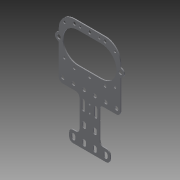
# Autodesk Inventor part: xcarriage
Saved by Autodesk Inventor 2014 (Build 180170000, 170)
## iProperties
Created: 2013-12-23
Part Number: xcarriage
Material: Generic
Document SubType Name: Modeling
Designer: stephen
Density: 1 g/cm^3
Appearance: Default
Author: stephen
Autodesk Inventor part; units mm, degrees
ref_plane "YZ Plane" through (0, 0, 0) normal (1, 0, 0) x (0, 1, 0)
ref_plane "XZ Plane" through (0, 0, 0) normal (0, 1, 0) x (-1, 0, 0)
ref_plane "XY Plane" through (0, 0, 0) normal (0, 0, 1) x (1, 0, 0)
sketch "Sketch1" plane through (0, 0, 0) normal (0, 1, 0) x (-1, 0, 0)
  line L0 (191.3405, 93.7812) -> (191.3405, 90.7812)
  circle A0 centre (230.8405, 152.2812) radius 2.5
  arc A1 (154.4119, 200.0727) -> (155.8405, 201.9894) centre (153.8405, 201.9894) ccw
  line L1 (200.3405, 110.7812) -> (200.3405, 113.7812)
  line L2 (186.3405, 90.7812) -> (186.3405, 93.7812)
  circle A2 centre (216.8405, 152.2812) radius 2.5
  arc A3 (213.8405, 145.2812) -> (208.8405, 140.2812) centre (213.8405, 140.2812) ccw
  line L3 (180.8405, 175.2812) -> (210.8405, 175.2812)
  arc A4 (182.8405, 127.2812) -> (182.8458, 127.0511) centre (187.8405, 127.2812) ccw
  line L4 (210.8405, 215.2812) -> (180.8405, 215.2812)
  arc A5 (201.8405, 129.2812) -> (205.8405, 129.2812) centre (203.8405, 129.2812) ccw
  arc A6 (154.4119, 200.0727) -> (154.4119, 190.4896) centre (155.8405, 195.2812) ccw
  line L5 (219.3405, 93.7812) -> (219.3405, 90.7812)
  line L6 (217.3405, 99.7812) -> (213.8405, 99.7812)
  arc A7 (214.3405, 90.7812) -> (219.3405, 90.7812) centre (216.8405, 90.7812) ccw
  line L7 (208.8405, 104.7812) -> (208.8405, 127.0511)
  arc A8 (200.3405, 110.7812) -> (205.3405, 110.7812) centre (202.8405, 110.7812) ccw
  circle A9 centre (215.8405, 220.2812) radius 2.1
  circle A10 centre (160.8405, 152.2812) radius 2.5
  arc A11 (191.3405, 93.7812) -> (186.3405, 93.7812) centre (188.8405, 93.7812) ccw
  line L8 (182.8405, 127.0511) -> (182.8405, 104.7812)
  arc A12 (169.3405, 89.7812) -> (174.3405, 84.7812) centre (174.3405, 89.7812) ccw
  circle A13 centre (215.8405, 170.2812) radius 2.1
  line L9 (175.8405, 225.2812) -> (215.8405, 225.2812)
  arc A14 (217.3405, 84.7812) -> (222.3405, 89.7812) centre (217.3405, 89.7812) ccw
  arc A15 (186.3405, 110.7812) -> (191.3405, 110.7812) centre (188.8405, 110.7812) ccw
  line L10 (205.3405, 93.7812) -> (205.3405, 90.7812)
  line L11 (186.3405, 110.7812) -> (186.3405, 113.7812)
  arc A16 (237.2691, 190.4896) -> (235.8405, 188.573) centre (237.8405, 188.573) ccw
  line L12 (177.3405, 93.7812) -> (177.3405, 90.7812)
  arc A17 (191.3405, 113.7812) -> (186.3405, 113.7812) centre (188.8405, 113.7812) ccw
  line L13 (189.8405, 129.2812) -> (189.8405, 139.2812)
  line L14 (235.8405, 188.573) -> (235.8405, 150.2812)
  circle A18 centre (175.8405, 170.2812) radius 2.1
  line L15 (172.3405, 90.7812) -> (172.3405, 93.7812)
  line L16 (174.3405, 84.7812) -> (217.3405, 84.7812)
  arc A19 (172.3405, 90.7812) -> (177.3405, 90.7812) centre (174.8405, 90.7812) ccw
  circle A20 centre (183.3405, 220.2812) radius 1.6
  line L17 (185.8405, 139.2812) -> (185.8405, 129.2812)
  arc A21 (222.3405, 94.7812) -> (217.3405, 99.7812) centre (217.3405, 94.7812) ccw
  arc A22 (200.3405, 90.7812) -> (205.3405, 90.7812) centre (202.8405, 90.7812) ccw
  line L18 (155.8405, 150.2812) -> (155.8405, 188.573)
  arc A23 (235.8405, 205.2812) -> (215.8405, 225.2812) centre (215.8405, 205.2812) ccw
  arc A24 (155.8405, 188.573) -> (154.4119, 190.4896) centre (153.8405, 188.573) ccw
  line L19 (222.3405, 89.7812) -> (222.3405, 94.7812)
  arc A25 (185.8405, 129.2812) -> (189.8405, 129.2812) centre (187.8405, 129.2812) ccw
  circle A26 centre (155.8405, 195.2812) radius 2.6
  line L20 (160.8405, 145.2812) -> (177.8405, 145.2812)
  arc A27 (177.3405, 93.7812) -> (172.3405, 93.7812) centre (174.8405, 93.7812) ccw
  arc A28 (186.3405, 90.7812) -> (191.3405, 90.7812) centre (188.8405, 90.7812) ccw
  circle A29 centre (202.8405, 152.2812) radius 2.5
  arc A30 (182.8405, 140.2812) -> (177.8405, 145.2812) centre (177.8405, 140.2812) ccw
  circle A31 centre (174.8405, 152.2812) radius 2.5
  line L21 (235.8405, 205.2812) -> (235.8405, 201.9894)
  line L22 (155.8405, 201.9894) -> (155.8405, 205.2812)
  line L23 (201.8405, 139.2812) -> (201.8405, 129.2812)
  circle A32 centre (162.8405, 215.2812) radius 1.75
  line L24 (208.8405, 127.0511) -> (208.8352, 127.0511)
  arc A33 (237.2691, 190.4896) -> (237.2691, 200.0727) centre (235.8405, 195.2812) ccw
  circle A34 centre (208.3405, 220.2812) radius 1.6
  arc A35 (208.8405, 104.7812) -> (213.8405, 99.7812) centre (213.8405, 104.7812) ccw
  arc A36 (189.8405, 139.2812) -> (185.8405, 139.2812) centre (187.8405, 139.2812) ccw
  arc A37 (219.3405, 93.7812) -> (214.3405, 93.7812) centre (216.8405, 93.7812) ccw
  line L25 (169.3405, 94.7812) -> (169.3405, 89.7812)
  circle A38 centre (228.8405, 175.2812) radius 1.75
  arc A39 (210.8405, 175.2812) -> (210.8405, 215.2812) centre (210.8405, 195.2812) ccw
  arc A40 (208.8352, 127.0511) -> (208.8405, 127.2812) centre (203.8405, 127.2812) ccw
  arc A41 (205.3405, 113.7812) -> (200.3405, 113.7812) centre (202.8405, 113.7812) ccw
  circle A42 centre (188.8405, 152.2812) radius 2.5
  arc A43 (174.3405, 99.7812) -> (169.3405, 94.7812) centre (174.3405, 94.7812) ccw
  circle A44 centre (195.8405, 220.2812) radius 2.1
  arc A45 (235.8405, 201.9894) -> (237.2691, 200.0727) centre (237.8405, 201.9894) ccw
  arc A46 (205.8405, 139.2812) -> (201.8405, 139.2812) centre (203.8405, 139.2812) ccw
  arc A47 (205.3405, 93.7812) -> (200.3405, 93.7812) centre (202.8405, 93.7812) ccw
  line L26 (208.8405, 127.2812) -> (208.8405, 140.2812)
  line L27 (182.8405, 127.2812) -> (182.8405, 140.2812)
  arc A48 (155.8405, 150.2812) -> (160.8405, 145.2812) centre (160.8405, 150.2812) ccw
  line L28 (200.3405, 90.7812) -> (200.3405, 93.7812)
  line L29 (182.8458, 127.0511) -> (182.8405, 127.0511)
  circle A49 centre (195.8405, 170.2812) radius 2.1
  arc A50 (180.8405, 215.2812) -> (180.8405, 175.2812) centre (180.8405, 195.2812) ccw
  line L30 (205.3405, 113.7812) -> (205.3405, 110.7812)
  line L31 (205.8405, 129.2812) -> (205.8405, 139.2812)
  line L32 (177.8405, 99.7812) -> (174.3405, 99.7812)
  circle A51 centre (235.8405, 195.2812) radius 2.6
  circle A52 centre (195.8405, 129.2812) radius 1.25
  line L33 (191.3405, 113.7812) -> (191.3405, 110.7812)
  arc A53 (175.8405, 225.2812) -> (155.8405, 205.2812) centre (175.8405, 205.2812) ccw
  circle A54 centre (162.8405, 175.2812) radius 1.75
  arc A55 (230.8405, 145.2812) -> (235.8405, 150.2812) centre (230.8405, 150.2812) ccw
  arc A56 (177.8405, 99.7812) -> (182.8405, 104.7812) centre (177.8405, 104.7812) ccw
  circle A57 centre (228.8405, 215.2812) radius 1.75
  circle A58 centre (175.8405, 220.2812) radius 2.1
  line L34 (213.8405, 145.2812) -> (230.8405, 145.2812)
  line L35 (214.3405, 90.7812) -> (214.3405, 93.7812)
  circle A59 centre (195.8405, 139.2812) radius 1.25
  line L36 (191.3405, 93.7812) -> (191.3405, 90.7812)
  circle A60 centre (230.8405, 152.2812) radius 2.5
  arc A61 (154.4119, 200.0727) -> (155.8405, 201.9894) centre (153.8405, 201.9894) ccw
  line L37 (200.3405, 110.7812) -> (200.3405, 113.7812)
  line L38 (186.3405, 90.7812) -> (186.3405, 93.7812)
  circle A62 centre (216.8405, 152.2812) radius 2.5
  arc A63 (213.8405, 145.2812) -> (208.8405, 140.2812) centre (213.8405, 140.2812) ccw
  line L39 (180.8405, 175.2812) -> (210.8405, 175.2812)
  arc A64 (182.8405, 127.2812) -> (182.8458, 127.0511) centre (187.8405, 127.2812) ccw
  line L40 (210.8405, 215.2812) -> (180.8405, 215.2812)
  arc A65 (201.8405, 129.2812) -> (205.8405, 129.2812) centre (203.8405, 129.2812) ccw
  arc A66 (154.4119, 200.0727) -> (154.4119, 190.4896) centre (155.8405, 195.2812) ccw
  line L41 (219.3405, 93.7812) -> (219.3405, 90.7812)
  line L42 (217.3405, 99.7812) -> (213.8405, 99.7812)
  arc A67 (214.3405, 90.7812) -> (219.3405, 90.7812) centre (216.8405, 90.7812) ccw
  line L43 (208.8405, 104.7812) -> (208.8405, 127.0511)
  arc A68 (200.3405, 110.7812) -> (205.3405, 110.7812) centre (202.8405, 110.7812) ccw
  circle A69 centre (215.8405, 220.2812) radius 2.1
  circle A70 centre (160.8405, 152.2812) radius 2.5
  arc A71 (191.3405, 93.7812) -> (186.3405, 93.7812) centre (188.8405, 93.7812) ccw
  line L44 (182.8405, 127.0511) -> (182.8405, 104.7812)
  arc A72 (169.3405, 89.7812) -> (174.3405, 84.7812) centre (174.3405, 89.7812) ccw
  circle A73 centre (215.8405, 170.2812) radius 2.1
  line L45 (175.8405, 225.2812) -> (215.8405, 225.2812)
  arc A74 (217.3405, 84.7812) -> (222.3405, 89.7812) centre (217.3405, 89.7812) ccw
  arc A75 (186.3405, 110.7812) -> (191.3405, 110.7812) centre (188.8405, 110.7812) ccw
  line L46 (205.3405, 93.7812) -> (205.3405, 90.7812)
  line L47 (186.3405, 110.7812) -> (186.3405, 113.7812)
  arc A76 (237.2691, 190.4896) -> (235.8405, 188.573) centre (237.8405, 188.573) ccw
  line L48 (177.3405, 93.7812) -> (177.3405, 90.7812)
  arc A77 (191.3405, 113.7812) -> (186.3405, 113.7812) centre (188.8405, 113.7812) ccw
  line L49 (189.8405, 129.2812) -> (189.8405, 139.2812)
  line L50 (235.8405, 188.573) -> (235.8405, 150.2812)
  circle A78 centre (175.8405, 170.2812) radius 2.1
  line L51 (172.3405, 90.7812) -> (172.3405, 93.7812)
  line L52 (174.3405, 84.7812) -> (217.3405, 84.7812)
  arc A79 (172.3405, 90.7812) -> (177.3405, 90.7812) centre (174.8405, 90.7812) ccw
  circle A80 centre (183.3405, 220.2812) radius 1.6
  line L53 (185.8405, 139.2812) -> (185.8405, 129.2812)
  arc A81 (222.3405, 94.7812) -> (217.3405, 99.7812) centre (217.3405, 94.7812) ccw
  arc A82 (200.3405, 90.7812) -> (205.3405, 90.7812) centre (202.8405, 90.7812) ccw
  line L54 (155.8405, 150.2812) -> (155.8405, 188.573)
  arc A83 (235.8405, 205.2812) -> (215.8405, 225.2812) centre (215.8405, 205.2812) ccw
  arc A84 (155.8405, 188.573) -> (154.4119, 190.4896) centre (153.8405, 188.573) ccw
  line L55 (222.3405, 89.7812) -> (222.3405, 94.7812)
  arc A85 (185.8405, 129.2812) -> (189.8405, 129.2812) centre (187.8405, 129.2812) ccw
  circle A86 centre (155.8405, 195.2812) radius 2.6
  line L56 (160.8405, 145.2812) -> (177.8405, 145.2812)
  arc A87 (177.3405, 93.7812) -> (172.3405, 93.7812) centre (174.8405, 93.7812) ccw
  arc A88 (186.3405, 90.7812) -> (191.3405, 90.7812) centre (188.8405, 90.7812) ccw
  circle A89 centre (202.8405, 152.2812) radius 2.5
  arc A90 (182.8405, 140.2812) -> (177.8405, 145.2812) centre (177.8405, 140.2812) ccw
  circle A91 centre (174.8405, 152.2812) radius 2.5
  line L57 (235.8405, 205.2812) -> (235.8405, 201.9894)
  line L58 (155.8405, 201.9894) -> (155.8405, 205.2812)
  line L59 (201.8405, 139.2812) -> (201.8405, 129.2812)
  circle A92 centre (162.8405, 215.2812) radius 1.75
  line L60 (208.8405, 127.0511) -> (208.8352, 127.0511)
  arc A93 (237.2691, 190.4896) -> (237.2691, 200.0727) centre (235.8405, 195.2812) ccw
  circle A94 centre (208.3405, 220.2812) radius 1.6
  arc A95 (208.8405, 104.7812) -> (213.8405, 99.7812) centre (213.8405, 104.7812) ccw
  arc A96 (189.8405, 139.2812) -> (185.8405, 139.2812) centre (187.8405, 139.2812) ccw
  arc A97 (219.3405, 93.7812) -> (214.3405, 93.7812) centre (216.8405, 93.7812) ccw
  line L61 (169.3405, 94.7812) -> (169.3405, 89.7812)
  circle A98 centre (228.8405, 175.2812) radius 1.75
  arc A99 (210.8405, 175.2812) -> (210.8405, 215.2812) centre (210.8405, 195.2812) ccw
  arc A100 (208.8352, 127.0511) -> (208.8405, 127.2812) centre (203.8405, 127.2812) ccw
  arc A101 (205.3405, 113.7812) -> (200.3405, 113.7812) centre (202.8405, 113.7812) ccw
  circle A102 centre (188.8405, 152.2812) radius 2.5
  arc A103 (174.3405, 99.7812) -> (169.3405, 94.7812) centre (174.3405, 94.7812) ccw
  circle A104 centre (195.8405, 220.2812) radius 2.1
  arc A105 (235.8405, 201.9894) -> (237.2691, 200.0727) centre (237.8405, 201.9894) ccw
  arc A106 (205.8405, 139.2812) -> (201.8405, 139.2812) centre (203.8405, 139.2812) ccw
  arc A107 (205.3405, 93.7812) -> (200.3405, 93.7812) centre (202.8405, 93.7812) ccw
  line L62 (208.8405, 127.2812) -> (208.8405, 140.2812)
  line L63 (182.8405, 127.2812) -> (182.8405, 140.2812)
  arc A108 (155.8405, 150.2812) -> (160.8405, 145.2812) centre (160.8405, 150.2812) ccw
  line L64 (200.3405, 90.7812) -> (200.3405, 93.7812)
  line L65 (182.8458, 127.0511) -> (182.8405, 127.0511)
  circle A109 centre (195.8405, 170.2812) radius 2.1
  arc A110 (180.8405, 215.2812) -> (180.8405, 175.2812) centre (180.8405, 195.2812) ccw
  line L66 (205.3405, 113.7812) -> (205.3405, 110.7812)
  line L67 (205.8405, 129.2812) -> (205.8405, 139.2812)
  line L68 (177.8405, 99.7812) -> (174.3405, 99.7812)
  circle A111 centre (235.8405, 195.2812) radius 2.6
  circle A112 centre (195.8405, 129.2812) radius 1.25
  line L69 (191.3405, 113.7812) -> (191.3405, 110.7812)
  arc A113 (175.8405, 225.2812) -> (155.8405, 205.2812) centre (175.8405, 205.2812) ccw
  circle A114 centre (162.8405, 175.2812) radius 1.75
  arc A115 (230.8405, 145.2812) -> (235.8405, 150.2812) centre (230.8405, 150.2812) ccw
  arc A116 (177.8405, 99.7812) -> (182.8405, 104.7812) centre (177.8405, 104.7812) ccw
  circle A117 centre (228.8405, 215.2812) radius 1.75
  circle A118 centre (175.8405, 220.2812) radius 2.1
  line L70 (213.8405, 145.2812) -> (230.8405, 145.2812)
  line L71 (214.3405, 90.7812) -> (214.3405, 93.7812)
  circle A119 centre (195.8405, 139.2812) radius 1.25
  line L72 (191.3405, 93.7812) -> (191.3405, 90.7812)
  circle A120 centre (230.8405, 152.2812) radius 2.5
  arc A121 (154.4119, 200.0727) -> (155.8405, 201.9894) centre (153.8405, 201.9894) ccw
  line L73 (200.3405, 110.7812) -> (200.3405, 113.7812)
  line L74 (186.3405, 90.7812) -> (186.3405, 93.7812)
  circle A122 centre (216.8405, 152.2812) radius 2.5
  arc A123 (213.8405, 145.2812) -> (208.8405, 140.2812) centre (213.8405, 140.2812) ccw
  line L75 (180.8405, 175.2812) -> (210.8405, 175.2812)
  arc A124 (182.8405, 127.2812) -> (182.8458, 127.0511) centre (187.8405, 127.2812) ccw
  line L76 (210.8405, 215.2812) -> (180.8405, 215.2812)
  arc A125 (201.8405, 129.2812) -> (205.8405, 129.2812) centre (203.8405, 129.2812) ccw
  arc A126 (154.4119, 200.0727) -> (154.4119, 190.4896) centre (155.8405, 195.2812) ccw
  line L77 (219.3405, 93.7812) -> (219.3405, 90.7812)
  line L78 (217.3405, 99.7812) -> (213.8405, 99.7812)
  arc A127 (214.3405, 90.7812) -> (219.3405, 90.7812) centre (216.8405, 90.7812) ccw
  line L79 (208.8405, 104.7812) -> (208.8405, 127.0511)
  arc A128 (200.3405, 110.7812) -> (205.3405, 110.7812) centre (202.8405, 110.7812) ccw
  circle A129 centre (215.8405, 220.2812) radius 2.1
  circle A130 centre (160.8405, 152.2812) radius 2.5
  arc A131 (191.3405, 93.7812) -> (186.3405, 93.7812) centre (188.8405, 93.7812) ccw
  line L80 (182.8405, 127.0511) -> (182.8405, 104.7812)
  arc A132 (169.3405, 89.7812) -> (174.3405, 84.7812) centre (174.3405, 89.7812) ccw
  circle A133 centre (215.8405, 170.2812) radius 2.1
  line L81 (175.8405, 225.2812) -> (215.8405, 225.2812)
  arc A134 (217.3405, 84.7812) -> (222.3405, 89.7812) centre (217.3405, 89.7812) ccw
  arc A135 (186.3405, 110.7812) -> (191.3405, 110.7812) centre (188.8405, 110.7812) ccw
  line L82 (205.3405, 93.7812) -> (205.3405, 90.7812)
  line L83 (186.3405, 110.7812) -> (186.3405, 113.7812)
  arc A136 (237.2691, 190.4896) -> (235.8405, 188.573) centre (237.8405, 188.573) ccw
  line L84 (177.3405, 93.7812) -> (177.3405, 90.7812)
  arc A137 (191.3405, 113.7812) -> (186.3405, 113.7812) centre (188.8405, 113.7812) ccw
  line L85 (189.8405, 129.2812) -> (189.8405, 139.2812)
  line L86 (235.8405, 188.573) -> (235.8405, 150.2812)
  circle A138 centre (175.8405, 170.2812) radius 2.1
  line L87 (172.3405, 90.7812) -> (172.3405, 93.7812)
  line L88 (174.3405, 84.7812) -> (217.3405, 84.7812)
  arc A139 (172.3405, 90.7812) -> (177.3405, 90.7812) centre (174.8405, 90.7812) ccw
  circle A140 centre (183.3405, 220.2812) radius 1.6
  line L89 (185.8405, 139.2812) -> (185.8405, 129.2812)
  arc A141 (222.3405, 94.7812) -> (217.3405, 99.7812) centre (217.3405, 94.7812) ccw
  arc A142 (200.3405, 90.7812) -> (205.3405, 90.7812) centre (202.8405, 90.7812) ccw
  line L90 (155.8405, 150.2812) -> (155.8405, 188.573)
  arc A143 (235.8405, 205.2812) -> (215.8405, 225.2812) centre (215.8405, 205.2812) ccw
  arc A144 (155.8405, 188.573) -> (154.4119, 190.4896) centre (153.8405, 188.573) ccw
  line L91 (222.3405, 89.7812) -> (222.3405, 94.7812)
  arc A145 (185.8405, 129.2812) -> (189.8405, 129.2812) centre (187.8405, 129.2812) ccw
  circle A146 centre (155.8405, 195.2812) radius 2.6
  line L92 (160.8405, 145.2812) -> (177.8405, 145.2812)
  arc A147 (177.3405, 93.7812) -> (172.3405, 93.7812) centre (174.8405, 93.7812) ccw
  arc A148 (186.3405, 90.7812) -> (191.3405, 90.7812) centre (188.8405, 90.7812) ccw
  circle A149 centre (202.8405, 152.2812) radius 2.5
  arc A150 (182.8405, 140.2812) -> (177.8405, 145.2812) centre (177.8405, 140.2812) ccw
  circle A151 centre (174.8405, 152.2812) radius 2.5
  line L93 (235.8405, 205.2812) -> (235.8405, 201.9894)
  line L94 (155.8405, 201.9894) -> (155.8405, 205.2812)
  line L95 (201.8405, 139.2812) -> (201.8405, 129.2812)
  circle A152 centre (162.8405, 215.2812) radius 1.75
  line L96 (208.8405, 127.0511) -> (208.8352, 127.0511)
  arc A153 (237.2691, 190.4896) -> (237.2691, 200.0727) centre (235.8405, 195.2812) ccw
  circle A154 centre (208.3405, 220.2812) radius 1.6
  arc A155 (208.8405, 104.7812) -> (213.8405, 99.7812) centre (213.8405, 104.7812) ccw
  arc A156 (189.8405, 139.2812) -> (185.8405, 139.2812) centre (187.8405, 139.2812) ccw
  arc A157 (219.3405, 93.7812) -> (214.3405, 93.7812) centre (216.8405, 93.7812) ccw
  line L97 (169.3405, 94.7812) -> (169.3405, 89.7812)
  circle A158 centre (228.8405, 175.2812) radius 1.75
  arc A159 (210.8405, 175.2812) -> (210.8405, 215.2812) centre (210.8405, 195.2812) ccw
  arc A160 (208.8352, 127.0511) -> (208.8405, 127.2812) centre (203.8405, 127.2812) ccw
  arc A161 (205.3405, 113.7812) -> (200.3405, 113.7812) centre (202.8405, 113.7812) ccw
  circle A162 centre (188.8405, 152.2812) radius 2.5
  arc A163 (174.3405, 99.7812) -> (169.3405, 94.7812) centre (174.3405, 94.7812) ccw
  circle A164 centre (195.8405, 220.2812) radius 2.1
  arc A165 (235.8405, 201.9894) -> (237.2691, 200.0727) centre (237.8405, 201.9894) ccw
  arc A166 (205.8405, 139.2812) -> (201.8405, 139.2812) centre (203.8405, 139.2812) ccw
  arc A167 (205.3405, 93.7812) -> (200.3405, 93.7812) centre (202.8405, 93.7812) ccw
  line L98 (208.8405, 127.2812) -> (208.8405, 140.2812)
  line L99 (182.8405, 127.2812) -> (182.8405, 140.2812)
  arc A168 (155.8405, 150.2812) -> (160.8405, 145.2812) centre (160.8405, 150.2812) ccw
  line L100 (200.3405, 90.7812) -> (200.3405, 93.7812)
  line L101 (182.8458, 127.0511) -> (182.8405, 127.0511)
  circle A169 centre (195.8405, 170.2812) radius 2.1
  arc A170 (180.8405, 215.2812) -> (180.8405, 175.2812) centre (180.8405, 195.2812) ccw
  line L102 (205.3405, 113.7812) -> (205.3405, 110.7812)
  line L103 (205.8405, 129.2812) -> (205.8405, 139.2812)
  line L104 (177.8405, 99.7812) -> (174.3405, 99.7812)
  circle A171 centre (235.8405, 195.2812) radius 2.6
  circle A172 centre (195.8405, 129.2812) radius 1.25
  line L105 (191.3405, 113.7812) -> (191.3405, 110.7812)
  arc A173 (175.8405, 225.2812) -> (155.8405, 205.2812) centre (175.8405, 205.2812) ccw
  circle A174 centre (162.8405, 175.2812) radius 1.75
  arc A175 (230.8405, 145.2812) -> (235.8405, 150.2812) centre (230.8405, 150.2812) ccw
  arc A176 (177.8405, 99.7812) -> (182.8405, 104.7812) centre (177.8405, 104.7812) ccw
  circle A177 centre (228.8405, 215.2812) radius 1.75
  circle A178 centre (175.8405, 220.2812) radius 2.1
  line L106 (213.8405, 145.2812) -> (230.8405, 145.2812)
  line L107 (214.3405, 90.7812) -> (214.3405, 93.7812)
  circle A179 centre (195.8405, 139.2812) radius 1.25
  point P0 (0, 0)
  constraints: 252 tangent, 228 point on circle, 216 end point, 180 centre point, 150 equal radius, 60 parallel, 21 perpendicular, 6 concentric, 3 collinear
extrude "Extrusion1" add sketch "Sketch1" along normal blind 1.25
body "Solid1"
